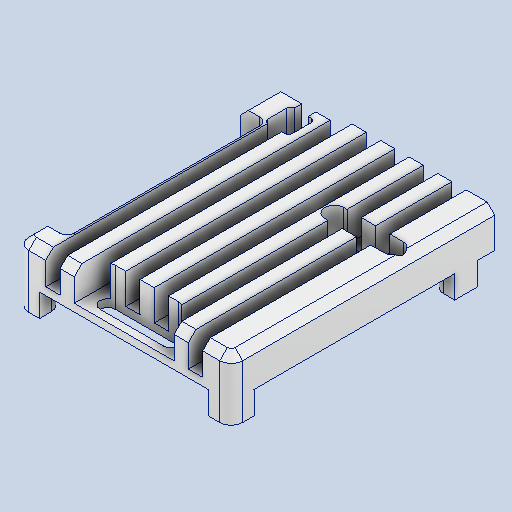
# Autodesk Inventor part: Raspberry-Pi-4B heatsink2
Saved by Autodesk Inventor 2023 (Build 270158000, 158)
## iProperties
Created: 2023-04-10
Part Number: Raspberry-Pi-4B heatsink2
Material: Aluminum 6061
Document SubType Name: Modeling
Designer: ASARe-DAQ-PC
Density: 2.7 g/cm^3
Appearance: Aluminum - Flat
Mass: 63.768 g
Surface Area: 166.404 cm^2
Volume: 23.6178 cm^3
Author: ASARe-DAQ-PC
Autodesk Inventor part; units mm, degrees
ref_plane "YZ Plane" through (0, 0, 0) normal (1, 0, 0) x (0, 1, 0)
ref_plane "XZ Plane" through (0, 0, 0) normal (0, 1, 0) x (-1, 0, 0)
ref_plane "XY Plane" through (0, 0, 0) normal (0, 0, 1) x (1, 0, 0)
sketch "Sketch1" plane through (0, 0, 0) normal (0, 1, 0) x (-1, 0, 0)
  line L0 (3, 0) -> (53, 0)
  line L1 (56, -3) -> (56, -82)
  line L2 (53, -85) -> (3, -85)
  line L3 (0, -82) -> (0, -3)
  arc A0 (56, -3) -> (53, 0) centre (53, -3) ccw
  arc A1 (53, -85) -> (56, -82) centre (53, -82) ccw
  arc A2 (0, -82) -> (3, -85) centre (3, -82) ccw
  arc A3 (3, 0) -> (0, -3) centre (3, -3) ccw
  point P0 (0, 0)
  point P1 (56, 0)
  point P2 (0, -85)
  dimension "d0" = 56
  dimension "d1" = 85
  dimension "d2" = 3
  constraints: 8 end point, 8 point on circle, 8 tangent, 6 point on line, 4 centre point, 3 equal radius, 2 parallel, 1 horizontal, 1 perpendicular
  measures "d0" distance of point (0, 0) point (56, 0)
  measures "d1" distance of point (0, -85) point (0, 0)
  measures "d2" radius of A0
extrude "Extrusion1" add sketch "Sketch1" along normal blind 10
chamfer "Chamfer1" distance 2 angle 45 8 edges at (0, 10, -42.5) (-0.8787, 10, -84.1213) (-28, 10, -85) (-55.1213, 10, -84.1213) (-56, 10, -42.5) (-55.1213, 10, -0.8787) (-28, 10, 0) (-0.8787, 10, -0.8787)
sketch "Sketch2" plane through (0, 0, 0) normal (0, 1, 0) x (-1, 0, 0)
  line L0 (53, 0) -> (3, 0) projected
  line L1 (3, -85) -> (53, -85) projected
  line L2 (44.8, 0) -> (48.5333, 0)
  line L3 (48.5333, 0) -> (48.5333, -85)
  line L4 (48.5333, -85) -> (44.8, -85)
  line L5 (44.8, -85) -> (44.8, 0)
  line L6 (56, -82) -> (56, -3) projected
  line L7 (41.0667, 0) -> (44.8, 0)
  line L8 (44.8, 0) -> (44.8, -85)
  line L9 (44.8, -85) -> (41.0667, -85)
  line L10 (41.0667, -85) -> (41.0667, 0)
  line L11 (37.3334, 0) -> (41.0667, 0)
  line L12 (41.0667, 0) -> (41.0667, -85)
  line L13 (41.0667, -85) -> (37.3334, -85)
  line L14 (37.3334, -85) -> (37.3334, 0)
  line L15 (33.6001, 0) -> (37.3334, 0)
  line L16 (37.3334, 0) -> (37.3334, -85)
  line L17 (37.3334, -85) -> (33.6001, -85)
  line L18 (33.6001, -85) -> (33.6001, 0)
  line L19 (29.8668, 0) -> (33.6001, 0)
  line L20 (33.6001, 0) -> (33.6001, -85)
  line L21 (33.6001, -85) -> (29.8668, -85)
  line L22 (29.8668, -85) -> (29.8668, 0)
  line L23 (26.1335, 0) -> (29.8668, 0)
  line L24 (29.8668, 0) -> (29.8668, -85)
  line L25 (29.8668, -85) -> (26.1335, -85)
  line L26 (26.1335, -85) -> (26.1335, 0)
  line L27 (22.4002, 0) -> (26.1335, 0)
  line L28 (26.1335, 0) -> (26.1335, -85)
  line L29 (26.1335, -85) -> (22.4002, -85)
  line L30 (22.4002, -85) -> (22.4002, 0)
  line L31 (18.6669, 0) -> (22.4002, 0)
  line L32 (22.4002, 0) -> (22.4002, -85)
  line L33 (22.4002, -85) -> (18.6669, -85)
  line L34 (18.6669, -85) -> (18.6669, 0)
  line L35 (14.9336, 0) -> (18.6669, 0)
  line L36 (18.6669, 0) -> (18.6669, -85)
  line L37 (18.6669, -85) -> (14.9336, -85)
  line L38 (14.9336, -85) -> (14.9336, 0)
  line L39 (11.2003, 0) -> (14.9336, 0)
  line L40 (14.9336, 0) -> (14.9336, -85)
  line L41 (14.9336, -85) -> (11.2003, -85)
  line L42 (11.2003, -85) -> (11.2003, 0)
  line L43 (7.467, 0) -> (11.2003, 0)
  line L44 (11.2003, 0) -> (11.2003, -85)
  line L45 (11.2003, -85) -> (7.467, -85)
  line L46 (7.467, -85) -> (7.467, 0)
  point P0 (0, 0)
  dimension "d8" = 7.4667
  dimension "d9" = 3.7333
  dimension "d12" = 3.7333
  constraints: 88 end point, 2 horizontal, 2 parallel, 2 point on line, 1 perpendicular, 80 other
  measures "d8" distance between parallel lines of L6 L3
  measures "d9" distance between parallel lines of L5 L3
  measures "d12" distance of L2.start L7.start
extrude "Extrusion2" cut sketch "Sketch2" against normal blind 8 from surface at 10 contours L3 L1 L5 L0 | L10 L1 L14 L0 | L18 L1 L22 L0 | L26 L1 L30 L0 | L34 L1 L38 L0 | L42 L1 L46 L0
sketch "Sketch3" plane through (0, 0, 0) normal (0, -1, 0) x (1, 0, 0)
  line L0 (-3, 0) -> (-5.85, 0)
  line L1 (-5.85, 0) -> (-5.85, -3)
  line L2 (-2.85, -6) -> (0, -6)
  line L3 (0, -6) -> (0, -3)
  line L4 (0, -3) -> (0, -82) projected
  line L5 (0, -58.5) -> (-1.425, -58.5)
  line L6 (-5.85, -64.5) -> (-5.85, -64.5)
  line L7 (-6.2545, -64.5) -> (0, -64.5)
  line L8 (0, -64.5) -> (0, -58.5)
  line L9 (-28, 0) -> (-28, -85) construction
  line L10 (-53, 0) -> (-3, 0) projected
  line L11 (-3, -85) -> (-53, -85) projected
  arc A0 (0, -3) -> (-3, 0) centre (-3, -3) ccw
  arc A1 (-5.85, -3) -> (-2.85, -6) centre (-2.85, -3) ccw
  line L12 (0, -6) -> (-5.85, -6)
  line L13 (0, -58.5) -> (-2.85, -58.5)
  line L14 (-2.85, -64.5) -> (0, -64.5)
  line L15 (-5.85, -61.5) -> (-5.85, -61.5)
  arc A2 (-2.85, -58.5) -> (-5.85, -61.5) centre (-2.85, -61.5) ccw
  arc A3 (-5.85, -61.5) -> (-2.85, -64.5) centre (-2.85, -61.5) ccw
  line L16 (0, -58.5) -> (-5.85, -58.5)
  line L17 (-5.85, -58.5) -> (-5.85, -64.5)
  line L18 (-5.85, -64.5) -> (0, -64.5)
  line L19 (0, -3) -> (0, -82) projected
  line L20 (-5.85, -6) -> (-5.85, 0)
  line L21 (-53, 0) -> (-50.15, 0)
  line L22 (-50.15, 0) -> (-50.15, -3)
  line L23 (-53.15, -6) -> (-56, -6)
  line L24 (-56, -6) -> (-56, -3)
  line L25 (-56, -58.5) -> (-54.575, -58.5)
  line L26 (-50.15, -64.5) -> (-50.15, -64.5)
  line L27 (-49.7455, -64.5) -> (-56, -64.5)
  line L28 (-56, -64.5) -> (-56, -58.5)
  arc A4 (-53, 0) -> (-56, -3) centre (-53, -3) ccw
  arc A5 (-53.15, -6) -> (-50.15, -3) centre (-53.15, -3) ccw
  line L29 (-56, -6) -> (-50.15, -6)
  line L30 (-56, -58.5) -> (-53.15, -58.5)
  line L31 (-53.15, -64.5) -> (-56, -64.5)
  line L32 (-50.15, -61.5) -> (-50.15, -61.5)
  arc A6 (-50.15, -61.5) -> (-53.15, -58.5) centre (-53.15, -61.5) ccw
  arc A7 (-53.15, -64.5) -> (-50.15, -61.5) centre (-53.15, -61.5) ccw
  line L33 (-56, -58.5) -> (-50.15, -58.5)
  line L34 (-50.15, -58.5) -> (-50.15, -64.5)
  line L35 (-50.15, -64.5) -> (-56, -64.5)
  line L36 (-50.15, -6) -> (-50.15, 0)
  point P0 (0, 0)
  point P1 (-0.7125, -58.5)
  point P2 (0, -64.5)
  point P3 (-56, 0)
  point P4 (-56, -3)
  point P5 (-53, 0)
  point P6 (-53.15, -58.5)
  point P7 (-5.85, -61.5)
  point P8 (-2.85, -64.5)
  point P9 (-5, -58.5)
  point P10 (-50.15, 0)
  point P11 (-5.717, -64.5)
  point P12 (-53.15, -64.5)
  point P13 (-53.15, -6)
  point P14 (-2.85, -6)
  point P15 (-2.85, -64.5)
  point P16 (-2.85, -58.5)
  point P17 (-53.15, -64.5)
  point P18 (-51, -58.5)
  point P19 (-5.85, -3)
  point P20 (-5.85, -61.5)
  point P21 (-5.85, -61.5)
  dimension "d19" = 6
  dimension "d21" = 58.5
  dimension "d22" = 6
  dimension "d25" = 28
  dimension "d26" = 3
  dimension "d29" = 3
  dimension "d30" = 3
  dimension "d56" = 5.85
  constraints: 66 end point, 26 symmetric about line, 25 point on line, 16 point on circle, 8 centre point, 8 tangent, 6 midpoint, 5 parallel, 3 perpendicular, 2 collinear, 2 horizontal, 1 concentric, 1 vertical, 4 other
  measures "d19" distance between parallel lines of L0 L2
  measures "d21" distance between parallel lines of L0 L5
  measures "d22" distance from line of point (-0.713, -58.5) L7
  measures "d25" distance between parallel lines of L4 L9
  measures "d26" radius of A0
  measures "d29" radius of A1
  measures "d30" radius of A2
  measures "d56" distance between parallel lines of L20 L4
extrude "Extrusion3" add sketch "Sketch3" along normal blind 6 contours A0 L3 L2 A1 L1 L0 | L4 L7 A3 A2 L13 L5 | L10 L22 A5 L23 L24 A4 | L25 L30 A6 A7 L27 L28
sketch "Sketch5" plane through (0, 0, 0) normal (0, -1, 0) x (1, 0, 0)
  line L0 (0, -64.5) -> (0, -82) projected
  line L1 (-56, -67) -> (-56, -85)
  line L2 (-56, -85) -> (0, -85)
  line L3 (0, -69) -> (-37, -69)
  line L4 (-38, -68) -> (-38, -68)
  line L5 (0, -85) -> (0, -69)
  line L6 (-39, -67) -> (-56, -67)
  line L7 (-22.4002, -85) -> (-22.4002, 0) projected
  line L8 (-3, -85) -> (-53, -85) projected
  line L9 (-56, -82) -> (-56, -64.5) projected
  line L10 (-50.15, 0) -> (-5.85, 0) projected
  line L11 (0, -6) -> (0, -82) projected
  line L12 (-44, -58) -> (-48.5, -58)
  line L13 (-49.5, -59) -> (-49.5, -64)
  line L14 (-43, -64) -> (-43, -59)
  line L15 (-4, -44) -> (-19.5, -44)
  line L16 (-19.5, -44) -> (-19.5, -49) construction
  line L17 (-19.5, -49) -> (-4, -49)
  line L18 (-4, -49) -> (-4, -44) construction
  arc A0 (-4, -49) -> (-4, -44) centre (-4, -46.5) ccw
  arc A1 (-19.5, -44) -> (-19.5, -49) centre (-19.5, -46.5) ccw
  line L19 (-56, -58.5) -> (-56, -6) projected
  line L20 (-19.7, -2) -> (-36.3, -2)
  line L21 (-36.3, -2) -> (-36.3, -6) construction
  line L22 (-36.3, -6) -> (-19.7, -6)
  line L23 (-19.7, -6) -> (-19.7, -2) construction
  arc A2 (-19.7, -6) -> (-19.7, -2) centre (-19.7, -4) ccw
  arc A3 (-36.3, -2) -> (-36.3, -6) centre (-36.3, -4) ccw
  arc A4 (-43, -59) -> (-44, -58) centre (-44, -59) ccw
  arc A5 (-44, -65) -> (-43, -64) centre (-44, -64) ccw
  arc A6 (-48.5, -58) -> (-49.5, -59) centre (-48.5, -59) ccw
  arc A7 (-49.5, -64) -> (-48.5, -65) centre (-48.5, -64) ccw
  arc A8 (-38, -68) -> (-37, -69) centre (-37, -68) ccw
  arc A9 (-38, -68) -> (-39, -67) centre (-39, -68) ccw
  line L24 (-44, -65) -> (-48.5, -65)
  line L25 (-56, -6) -> (-51, -6)
  line L26 (-49, -8) -> (-49, -56.5)
  line L27 (-51, -58.5) -> (-56, -58.5)
  line L28 (-56, -58.5) -> (-56, -6)
  arc A10 (-49, -8) -> (-51, -6) centre (-51, -8) ccw
  arc A11 (-51, -58.5) -> (-49, -56.5) centre (-51, -56.5) ccw
  point P0 (0, 0)
  point P1 (-38, -67)
  point P2 (-38, -69)
  point P3 (-38, -68)
  point P4 (-18.5, -69)
  point P5 (-43, -58)
  point P6 (-49.5, -58)
  point P7 (-22.4002, -6)
  point P8 (-22.4002, -2)
  point P9 (-22.4002, -69)
  point P10 (-22.4002, -45.8008)
  point P11 (-22.4002, -47.1992)
  dimension "d51" = 18
  dimension "d52" = 67
  dimension "d54" = 69
  dimension "d62" = 5
  dimension "d63" = 15.5
  dimension "d65" = 44
  dimension "d67" = 4
  dimension "d68" = 2
  dimension "d69" = 19.7
  dimension "d70" = 19.7
  dimension "d73" = 1
  dimension "d74" = 1
  dimension "d92" = 6.5
  dimension "d93" = 13
  dimension "d94" = 7
  dimension "d95" = 4
  dimension "d96" = 7
  dimension "d97" = 2
  dimension "d98" = 58
  constraints: 44 end point, 24 point on circle, 16 tangent, 12 centre point, 12 point on line, 8 parallel, 7 horizontal, 6 midpoint, 6 perpendicular, 5 equal radius, 1 vertical
  measures "d51" distance from line of point (-38, -68) L1
  measures "d52" distance between parallel lines of L10 L6
  measures "d54" distance from line of point (-18.5, -69) L10
  measures "d62" distance between parallel lines of L15 L17
  measures "d63" distance between parallel lines of L16 L18
  measures "d65" distance between parallel lines of L15 L10
  measures "d67" distance of L20.end L21.end
  measures "d68" distance between parallel lines of L10 L20
  measures "d69" distance between parallel lines of L11 L23
  measures "d70" distance between parallel lines of L19 L21
  measures "d73" radius of A4
  measures "d74" radius of A9
  measures "d92" distance between parallel lines of L9 L13
  measures "d93" distance between parallel lines of L9 L14
  measures "d94" distance between parallel lines of L12 L24
  measures "d95" distance between parallel lines of L11 L18
  measures "d96" distance between parallel lines of L19 L26
  measures "d97" radius of A10
  measures "d98" distance between parallel lines of L12 L10
extrude "Extrusion5" cut sketch "Sketch5" against normal through all
sketch "Sketch6" plane through (-41.0667, 2, 0) normal (0, 1, 0) x (1, 0, 0)
  line L0 (3.7333, 0) -> (7.4666, 0) projected
  line L1 (7.4666, 0) -> (7.4666, 2) projected
  line L2 (7.4666, 2) -> (4.7667, 2) projected
  line L3 (4.7667, 2) -> (3.7333, 2) projected
  line L4 (3.7333, 2) -> (3.7333, 0) projected
  line L5 (3.7333, 0) -> (7.4666, 0) projected
  line L6 (11.1999, 2) -> (11.1999, 0) projected
  line L7 (11.1999, 0) -> (14.9332, 0) projected
  line L8 (14.9332, 0) -> (14.9332, 2) projected
  line L9 (14.9332, 2) -> (11.1999, 2) projected
  line L10 (18.6665, 2) -> (18.6665, 0) projected
  line L11 (18.6665, 0) -> (22.3998, 0) projected
  line L12 (22.3998, 0) -> (22.3998, 2) projected
  line L13 (22.3998, 2) -> (21.3667, 2) projected
  line L14 (21.3667, 2) -> (18.6665, 2) projected
  arc A0 (21.3667, 2) -> (22.3998, 2.2875) centre (21.3667, 4) ccw projected
  line L15 (22.3998, 2) -> (21.3667, 2) projected
  line L16 (22.3998, 2) -> (22.3998, 2.2875) projected
  arc A1 (3.7333, 2.2877) -> (4.7667, 2) centre (4.7667, 4) ccw projected
  line L17 (3.7333, 2.2877) -> (3.7333, 2) projected
  line L18 (4.7667, 2) -> (3.7333, 2) projected
  point P0 (41.0667, 0)
extrude "Extrusion6" cut sketch "Sketch6" along normal blind 10
sketch "Sketch7" plane through (0, -6, 0) normal (0, -1, 0) x (1, 0, 0)
  line L0 (0, -6) -> (0, -3) projected
  line L1 (-3, 0) -> (-5.85, 0) projected
  line L2 (-56, -6) -> (-53.15, -6) projected
  line L3 (-50.15, 0) -> (-53, 0) projected
  line L4 (-56, -3) -> (-56, -6) projected
  line L5 (0, -64.5) -> (0, -58.5) projected
  line L6 (-56, -58.5) -> (-56, -64.5) projected
  point P0 (-3.5, -3.5)
  point P1 (-3.5, -61.5)
  point P2 (-52.5, -61.5)
  point P3 (-52.5, -3.5)
  point P4 (0, -61.5)
  point P5 (-56, -61.5)
  dimension "d84" = 3.5
  dimension "d85" = 3.5
  dimension "d87" = 3.5
  dimension "d88" = 3.5
  dimension "d90" = 3.5
  dimension "d91" = 3.5
  constraints: 2 horizontal alignment, 2 midpoint
  measures "d84" distance from line of L0 point (-3.5, -3.5)
  measures "d85" distance from line of L1 point (-3.5, -3.5)
  measures "d87" distance from line of L3 point (-52.5, -3.5)
  measures "d88" distance from line of L4 point (-52.5, -3.5)
  measures "d90" distance from line of point (-3.5, -61.5) L5
  measures "d91" distance from line of L6 point (-52.5, -61.5)
hole "Hole2" at (-3.5, -6, -3.5) at (-3.5, -6, -61.5) at (-52.5, -6, -61.5) at (-52.5, -6, -3.5) direction (0, 1, 0) diameter 2.1129 depth 7.8 tip angle 118 thread size "M2.6x0.45" class "6H" standard "ISO Metric profile"
sketch "Sketch8" plane through (0, 0, 0) normal (0, -1, 0) x (1, 0, 0)
  line L0 (-24.5147, -21.5082) -> (-40.7037, -21.5082)
  line L1 (-40.7037, -21.5082) -> (-40.7037, -37.0364)
  line L2 (-40.7037, -37.0364) -> (-24.5147, -37.0364)
  line L3 (-24.5147, -37.0364) -> (-24.5147, -21.5082)
  line L4 (-24.5147, -39.6134) -> (-40.2411, -39.6134)
  line L5 (-40.2411, -39.6134) -> (-40.2411, -51.8377)
  line L6 (-40.2411, -51.8377) -> (-24.5147, -51.8377)
  line L7 (-24.5147, -51.8377) -> (-24.5147, -39.6134)
  line L8 (-19.0303, -54.8112) -> (-28.9419, -54.8112)
  line L9 (-28.9419, -54.8112) -> (-28.9419, -65.1854)
  line L10 (-28.9419, -65.1854) -> (-19.0303, -65.1854)
  line L11 (-19.0303, -65.1854) -> (-19.0303, -54.8112)
  point P0 (0, 0)
  constraints: 24 end point, 6 parallel, 3 horizontal, 3 perpendicular, 1 point on line
extrude "Extrusion7" add sketch "Sketch8" along normal blind 4.5
body "Solid1"
